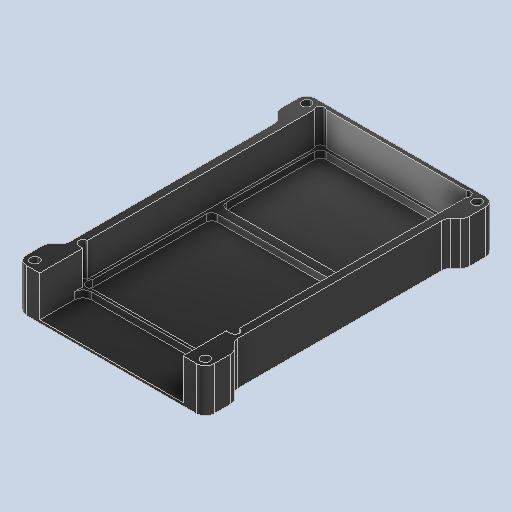
# Autodesk Inventor part: DK-42688-P_Cover
Saved by Autodesk Inventor 2024.2 (Build 282272000, 272)
## iProperties
Created: 2024-02-11
Part Number: DK-42688-P_Cover
Material: Aluminum 7075
Document SubType Name: Modeling
Designer: Masato Kubotera
Density: 2.81 g/cm^3
Appearance: Glossy - Black
Vendor: meviy
Author: Masato Kubotera
Autodesk Inventor part; units mm, degrees
ref_plane "XZ Plane" through (0, 0, 0) normal (0, 1, 0) x (-1, 0, 0)
ref_plane "XY Plane" through (0, 0, 0) normal (0, 0, 1) x (1, 0, 0)
derived "TorsoPelvisLowerFrame.ipt"
sketch "Sketch1" plane through (0, 0, 0) normal (0, 0, 1) x (1, 0, 0)
  line L0 (-50, -90) -> (50, -90)
  line L1 (50, -90) -> (50, 90)
  line L2 (50, 90) -> (-50, 90)
  line L3 (-50, 90) -> (-50, -90)
  line L4 (-50, -90) -> (50, 90) construction
  line L5 (50, -90) -> (-50, 90) construction
  line L6 (-50, 0) -> (50, 0)
  line L7 (0, -90) -> (0, 90) construction
  circle A0 centre (0, 55) radius 18.75
  circle A1 centre (0, -55) radius 18.75
  line L8 (0, 55) -> (24.75, 55) construction
  circle A2 centre (0, 55) radius 29 construction
  line L9 (-31, 39) -> (12, 39) construction
  line L10 (12, 39) -> (12, 71) construction
  line L11 (12, 71) -> (-31, 71) construction
  line L12 (-31, 71) -> (-31, 39) construction
  line L13 (-31, 39) -> (12, 71) construction
  line L14 (12, 39) -> (-31, 71) construction
  line L15 (-28, 41.5) -> (-1, 41.5) construction
  line L16 (-1, 41.5) -> (-1, 68.5) construction
  line L17 (-1, 68.5) -> (-28, 68.5) construction
  line L18 (-28, 68.5) -> (-28, 41.5) construction
  line L19 (-28, 41.5) -> (-1, 68.5) construction
  line L20 (-1, 41.5) -> (-28, 68.5) construction
  line L21 (-9.6933, 38.95) -> (-31, 38.95)
  line L22 (-31, 38.95) -> (-31, 71.05)
  line L23 (-31, 71.05) -> (-9.6933, 71.05)
  line L24 (11, 90) -> (11, 85) construction
  line L25 (38, 85) -> (38, 90) construction
  line L26 (50, 87.5) -> (-50, 87.5) construction
  line L27 (10.95, 90) -> (10.95, 85)
  line L28 (38.05, 85) -> (38.05, 90)
  line L29 (24.5, 85) -> (24.5, 90) construction
  line L30 (10.95, 85) -> (38.05, 85)
  line L31 (-10.95, 90) -> (-10.95, 85)
  line L32 (-11, 90) -> (-11, 85) construction
  line L33 (-24.5, 85) -> (-24.5, 90) construction
  line L34 (-10.95, 85) -> (-38.05, 85)
  line L35 (-38, 85) -> (-38, 90) construction
  line L36 (-38.05, 85) -> (-38.05, 90)
  arc A3 (35.05, 85) -> (38.05, 85) centre (36.55, 85) ccw
  arc A4 (10.95, 85) -> (13.95, 85) centre (12.45, 85) ccw
  arc A5 (-13.95, 85) -> (-10.95, 85) centre (-12.45, 85) ccw
  arc A6 (-38.05, 85) -> (-35.05, 85) centre (-36.55, 85) ccw
  line L37 (38.9, 39) -> (50.8, 39) construction
  line L38 (50.8, 39) -> (50.8, 64) construction
  line L39 (50.8, 64) -> (38.9, 64) construction
  line L40 (38.9, 64) -> (38.9, 39) construction
  line L41 (38.9, 39) -> (50.8, 64) construction
  line L42 (50.8, 39) -> (38.9, 64) construction
  line L43 (42.9, 39) -> (42.9, 64) construction
  line L44 (45, 64) -> (45, 39) construction
  line L45 (38.9, -64) -> (38.9, -39) construction
  line L46 (38.9, -39) -> (50.8, -39) construction
  line L47 (50.8, -39) -> (50.8, -64) construction
  line L48 (50.8, -64) -> (38.9, -64) construction
  line L49 (50, 38) -> (44.9, 38)
  line L50 (44.9, 38) -> (44.9, 65)
  line L51 (44.9, 65) -> (50, 65)
  arc A7 (44.9, 41) -> (44.9, 38) centre (44.9, 39.5) ccw
  arc A8 (44.9, 65) -> (44.9, 62) centre (44.9, 63.5) ccw
  line L52 (17.5, 54) -> (39.5, 54) construction
  line L53 (39.5, 54) -> (39.5, -54) construction
  line L54 (39.5, -54) -> (17.5, -54) construction
  line L55 (17.5, -54) -> (17.5, 54) construction
  line L56 (17.5, 54) -> (39.5, -54) construction
  line L57 (39.5, 54) -> (17.5, -54) construction
  line L58 (-44, -35) -> (6, -35) construction
  line L59 (6, -35) -> (6, 35) construction
  line L60 (6, 35) -> (-44, 35) construction
  line L61 (-44, 35) -> (-44, -35) construction
  line L62 (-44, -35) -> (6, 35) construction
  line L63 (6, -35) -> (-44, 35) construction
  line L64 (-40.5, -28) -> (2.5, -28) construction
  line L65 (2.5, -28) -> (2.5, 28) construction
  line L66 (2.5, 28) -> (-40.5, 28) construction
  line L67 (-40.5, 28) -> (-40.5, -28) construction
  line L68 (-40.5, -28) -> (2.5, 28) construction
  line L69 (2.5, -28) -> (-40.5, 28) construction
  line L70 (-41, 0) -> (-41, 24.0314)
  arc A9 (-41, 24.0314) -> (-40.5, 32) centre (-40.5, 28) ccw
  line L71 (-19, 35) -> (-19, -35) construction
  line L72 (3, 0) -> (3, 24.0314)
  line L73 (-44.1, -35.14) -> (6.1, 35.14) construction
  line L74 (38.9, 51.5) -> (50.8, 51.5) construction
  line L75 (50, 77.55) -> (45, 77.55)
  line L76 (45, 77.55) -> (45, 69.45)
  line L77 (45, 69.45) -> (50, 69.45)
  arc A10 (45, 71.5713) -> (47.1213, 69.45) centre (46.0607, 70.5107) ccw
  line L78 (45, 73.5) -> (50, 73.5) construction
  line L79 (50, 69.5) -> (45, 69.5) construction
  line L80 (45, 69.5) -> (45, 77.5) construction
  line L81 (45, 77.5) -> (50, 77.5) construction
  arc A11 (47.1213, 77.55) -> (45, 75.4287) centre (46.0607, 76.4893) ccw
  line L82 (-45, 69.45) -> (-50, 69.45)
  arc A12 (-47.1213, 69.45) -> (-45, 71.5713) centre (-46.0607, 70.5107) ccw
  line L83 (-45, 77.55) -> (-45, 69.45)
  arc A13 (-45, 75.4287) -> (-47.1213, 77.55) centre (-46.0607, 76.4893) ccw
  line L84 (-50, 77.55) -> (-45, 77.55)
  line L85 (38.9, -51.5) -> (50.8, -51.5) construction
  line L86 (22.05, 29) -> (22.05, -29)
  line L87 (44, -29) -> (44, 29)
  line L88 (44, 29) -> (22.05, 29)
  line L89 (21, 35) -> (39, 35)
  line L90 (39, 35) -> (39, 75)
  line L91 (39, 75) -> (21, 75)
  arc A14 (21, 35) -> (21, 75) centre (0, 55) ccw
  line L92 (12.5, 10) -> (17.5, 10) construction
  line L93 (17.5, 10) -> (17.5, 20) construction
  line L94 (17.5, 20) -> (12.5, 20) construction
  line L95 (12.5, 20) -> (12.5, 10) construction
  line L96 (12.5, 10) -> (17.5, 20) construction
  line L97 (17.5, 10) -> (12.5, 20) construction
  line L98 (17.55, 20.05) -> (12.45, 20.05)
  line L99 (12.45, 20.05) -> (12.45, 9.95)
  line L100 (12.45, 9.95) -> (17.55, 9.95)
  line L101 (17.55, 9.95) -> (17.55, 20.05)
  line L102 (17.55, 20.05) -> (12.45, 9.95) construction
  line L103 (12.45, 20.05) -> (17.55, 9.95) construction
  arc A15 (12.45, 12.95) -> (12.45, 9.95) centre (12.45, 11.45) ccw
  line L104 (15, 9.95) -> (15, 20.05) construction
  line L105 (12.45, 15) -> (17.55, 15) construction
  arc A16 (17.55, 9.95) -> (17.55, 12.95) centre (17.55, 11.45) ccw
  arc A17 (12.45, 20.05) -> (12.45, 17.05) centre (12.45, 18.55) ccw
  arc A18 (17.55, 17.05) -> (17.55, 20.05) centre (17.55, 18.55) ccw
  line L106 (44, -29) -> (22.05, -29)
  line L107 (50, 32.5) -> (-50, 32.5) construction
  line L108 (-50, 32.5) -> (-50, -32.5) construction
  line L109 (-50, -32.5) -> (50, -32.5) construction
  line L110 (50, -32.5) -> (50, 32.5) construction
  line L111 (50, 32.5) -> (-50, -32.5) construction
  line L112 (-50, 32.5) -> (50, -32.5) construction
  circle A19 centre (47, 29.5) radius 3 construction
  circle A20 centre (47, 29.5) radius 1.6 construction
  circle A21 centre (-47, 29.5) radius 1.6 construction
  circle A22 centre (-47, 29.5) radius 3 construction
  arc A23 (-17.6635, 32) -> (-0.9735, 26.0163) centre (0, 55) ccw
  line L113 (-40.5, 32) -> (-17.6635, 32)
  arc A24 (-0.9735, 26.0163) -> (3, 24.0314) centre (2.5, 28) ccw
  line L114 (-33, 71.05) -> (-42.5607, 71.05)
  line L115 (-42.5607, 71.05) -> (-42.5607, 38.95)
  line L116 (-42.5607, 38.95) -> (-33, 38.95)
  line L117 (-33, 38.95) -> (-33, 71.05)
  line L118 (-33, 71.05) -> (-42.5607, 38.95) construction
  line L119 (-42.5607, 71.05) -> (-33, 38.95) construction
  point P0 (0, 0)
  point P1 (12.375, 76.4341)
  point P2 (-12.375, 76.4341)
  point P3 (-24.75, 55)
  point P4 (-12.375, 33.5659)
  point P5 (12.375, 33.5659)
  point P6 (-9.5, 55)
  point P7 (-14.5, 55)
  point P8 (45.5, 87.5)
  point P9 (0, 87.5)
  point P10 (-45.5, 87.5)
  point P11 (44.85, 51.5)
  point P12 (42.9, 43.5)
  point P13 (42.9, 59.5)
  point P14 (28.5, 0)
  point P15 (-19, 0)
  point P16 (-19, 0)
  point P17 (15, 15)
  point P18 (15, 26)
  point P19 (-37.7803, 55)
sketch "Sketch2" plane through (0, 0, 0) normal (0, 0, 1) x (1, 0, 0)
  line L0 (-50, 0) -> (50, 0) construction
  line L1 (-34.55, 25.781) -> (48, 25.781) construction
  line L2 (48, 25.781) -> (48, -25.781) construction
  line L3 (48, -25.781) -> (-34.55, -25.781) construction
  line L4 (-34.55, -25.781) -> (-34.55, 25.781) construction
  line L5 (-34.55, 25.781) -> (48, -25.781) construction
  line L6 (48, 25.781) -> (-34.55, -25.781) construction
  line L7 (-35.05, -26.281) -> (48.5, -26.281)
  line L8 (48.5, -26.281) -> (48.5, 26.281)
  line L9 (48.5, 26.281) -> (-35.05, 26.281)
  line L10 (-35.05, 26.281) -> (-35.05, -26.281)
  line L11 (-35.05, -26.281) -> (48.5, 26.281) construction
  line L12 (48.5, -26.281) -> (-35.05, 26.281) construction
  line L13 (6.725, 25.781) -> (6.725, -25.781) construction
  line L14 (-35.05, -24.781) -> (-50, -24.781)
  circle A0 centre (-47, 29.5) radius 3 construction
  circle A1 centre (-47, 29.5) radius 1.6 construction
  circle A2 centre (47, 29.5) radius 3 construction
  circle A3 centre (47, 29.5) radius 1.6 construction
  line L15 (50, -32.5) -> (50, 32.5) projected
  line L16 (50, 32.5) -> (-50, 32.5) projected
  line L17 (-50, -32.5) -> (50, -32.5) projected
  line L18 (-50, 32.5) -> (-50, -32.5) projected
  line L19 (-34.05, 25.281) -> (-34.05, -25.281)
  line L20 (47.5, -23.281) -> (47.5, 23.281)
  arc A4 (45.5, -25.281) -> (47.5, -23.281) centre (45.5, -23.281) ccw
  arc A5 (47.5, 23.281) -> (45.5, 25.281) centre (45.5, 23.281) ccw
  line L21 (13, 23.281) -> (13, -23.281)
  line L22 (10, -23.281) -> (10, 23.281)
  line L23 (45.5, 25.281) -> (15, 25.281)
  line L24 (8, 25.281) -> (-34.05, 25.281)
  line L25 (-34.05, -25.281) -> (8, -25.281)
  line L26 (15, -25.281) -> (45.5, -25.281)
  arc A6 (13, -23.281) -> (15, -25.281) centre (15, -23.281) ccw
  arc A7 (15, 25.281) -> (13, 23.281) centre (15, 23.281) ccw
  arc A8 (10, 23.281) -> (8, 25.281) centre (8, 23.281) ccw
  arc A9 (8, -25.281) -> (10, -23.281) centre (8, -23.281) ccw
  arc A10 (46.3787, -26.281) -> (48.5, -24.1597) centre (47.4393, -25.2203) ccw
  arc A11 (48.5, 24.1597) -> (46.3787, 26.281) centre (47.4393, 25.2203) ccw
  line L27 (-35.05, 24.781) -> (-50, 24.781)
  arc A12 (-32.05, 26.281) -> (-35.05, 26.281) centre (-33.55, 26.281) ccw
  arc A13 (-35.05, -26.281) -> (-32.05, -26.281) centre (-33.55, -26.281) ccw
  line L28 (40, 32.5) -> (36.5, 29)
  line L29 (36.5, 29) -> (-36.5, 29)
  line L30 (-36.5, 29) -> (-40, 32.5)
  line L31 (0, -126) -> (0, 126) projected
  line L32 (40, -32.5) -> (36.5, -29)
  line L33 (36.5, -29) -> (-36.5, -29)
  line L34 (-36.5, -29) -> (-40, -32.5)
  arc A14 (-34.05, -22.4526) -> (-31.2216, -25.281) centre (-32.6358, -23.8668) ccw
  arc A15 (-31.2216, 25.281) -> (-34.05, 22.4526) centre (-32.6358, 23.8668) ccw
  point P0 (6.725, 0)
  point P1 (0, 0)
  point P2 (6.725, 0)
  point P3 (-37.075, -23.3995)
  point P4 (-47, -29.5)
  point P5 (47, -29.5)
  point P6 (46.3787, 26.281)
  point P7 (48.5, 24.1597)
  point P8 (-47.5, -24.781)
  point P9 (-40, -32.5)
  point P10 (40, -32.5)
  point P11 (0, -29)
  point P12 (0, -32.5)
  point P13 (-34.05, 22.4526)
  point P14 (-31.2216, 25.281)
  dimension "d1" = 82.55
  dimension "d2" = 51.562
  dimension "d3" = 0.5
  dimension "d4" = 0.5
  dimension "d23" = 1
  dimension "d25" = 2
  dimension "d32" = 35
  dimension "d33" = 38
  dimension "d35" = 1
  dimension "d36" = 2
  dimension "d38" = 1.5
  dimension "d39" = 1
  dimension "d40" = 135
  dimension "d41" = 58
  dimension "d42" = 10
  constraints: 60 end point, 27 point on circle, 16 symmetric about line, 14 tangent, 12 centre point, 9 parallel, 9 point on line, 8 midpoint, 7 equal radius, 6 horizontal, 4 perpendicular, 3 vertical, 10 other
  measures "d1" distance of L2.end L3.end
  measures "d2" distance of L1.end L2.end
  measures "d3" distance between parallel lines of L9 L1
  measures "d4" distance between parallel lines of L4 L10
  measures "d23" distance between parallel lines of L8 L20
  measures "d25" radius of A4
  measures "d32" distance between parallel lines of L21 L2
  measures "d33" distance between parallel lines of L22 L2
  measures "d35" distance between parallel lines of L9 L23
  measures "d36" distance between parallel lines of L2 L15
  measures "d38" radius of A11
  measures "d39" distance between parallel lines of L14 L3
  measures "d40" angle to the sketch x axis of L28
  measures "d41" distance between parallel lines of L33 L29
  measures "d42" distance of L28.start L15.end
extrude "Extrusion1" add sketch "Sketch2" along normal blind 1 contours L10 L9 L31 L24 A15 L19 A14 L25 L7 | A13 L7 L31 L33 L34 L17 L18 L14 L10 | L7 A13 | L14 L18 L27 L10 | L31 L25 A9 L22 A8 L24 L9 L8 L7 | L7 A10 L8 A11 L9 L31 L29 L28 L16 L15 L17 L32 L33 | L27 L18 L16 L30 L29 L31 L9 A12 L10 | L7 A10 | L31 L24 A8 L22 A9 L25 | L25 L19 L24 L31 | A12 L9 | L8 A10 | A14 L25 | A14 L19 | L24 A15 | L8 A11 | L19 A15 | A11 L9 | A4 L26 A6 L21 A7 L23 A5 L20
extrude "Extrusion2" add sketch "Sketch2" along normal blind 15 contours A13 L7 L31 L33 L34 L17 L18 L14 L10 | L7 A10 L8 A11 L9 L31 L29 L28 L16 L15 L17 L32 L33 | L27 L18 L16 L30 L29 L31 L9 A12 L10
extrude "Extrusion3" add sketch "Sketch2" along normal blind 3.4 contours L10 L9 L31 L24 A15 L19 A14 L25 L7 | L7 A13 | L31 L25 A9 L22 A8 L24 L9 L8 L7 | L7 A10 | A12 L9 | L8 A10 | L8 A11 | A11 L9
hole "Hole1" at (47, -29.5, 0) at (47, 29.5, 0) at (-47, -29.5, 0) at (-47, 29.5, 0) direction (0, 0, 1) diameter 3.2 end through all
fillet "Fillet1" radius 3 14 edges at (50, -32.5, 7.5) (50, 32.5, 7.5) (-50, -32.5, 7.5) (-50, 32.5, 7.5) (-40, -32.5, 7.5) (-40, 32.5, 7.5) (-36.5, 29, 7.5) (36.5, 29, 7.5) (40, 32.5, 7.5) (36.5, -29, 7.5) (40, -32.5, 7.5) (-36.5, -29, 7.5) (-35.05, 24.781, 2.2) (-35.05, -24.781, 2.2)
ref_plane "Work Plane1" through (6.725, -25.781, 0) normal (1, 0, 0) x (0, 1, 0)
equation "\"d35\" = d23"
equation "\"d24\" = d23"
body "Solid1"
